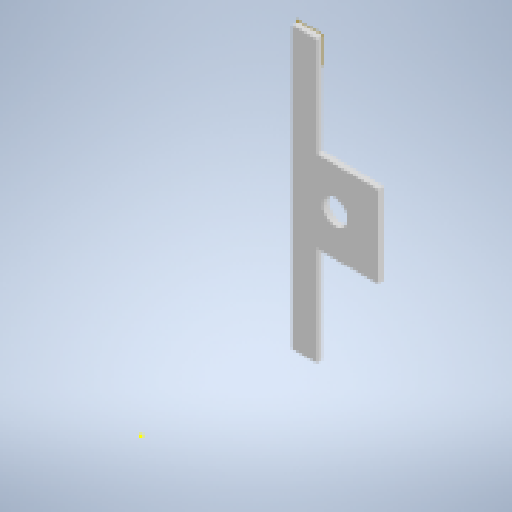
# Autodesk Inventor part: Linear rod connecting plate
Saved by Autodesk Inventor 2023.1 (Build 271208000, 208)
## iProperties
Created: 2023-02-01
Part Number: Linear rod connecting plate
Material: Generic
Document SubType Name: Modeling
Designer: dmargari
Density: 1 g/cm^3
Appearance: Default
Author: dmargari
Autodesk Inventor part; units mm, degrees
ref_plane "YZ Plane" through (0, 0, 0) normal (1, 0, 0) x (0, 1, 0)
ref_plane "XZ Plane" through (0, 0, 0) normal (0, 1, 0) x (-1, 0, 0)
ref_plane "XY Plane" through (0, 0, 0) normal (0, 0, 1) x (1, 0, 0)
sketch "Sketch1" plane through (0, 0, 0) normal (0, 0, 1) x (1, 0, 0)
  point P0 (0, 0)
ref_plane "Work Plane1" through (0, 125.1054, -82.3097) normal (0, 0, 1) x (1, 0, 0)
sketch "Sketch2" plane through (0, 125.1054, -82.3097) normal (0, 0, 1) x (1, 0, 0)
  circle A0 centre (0.3907, 0.2373) radius 6 projected
  circle A1 centre (0.3907, -124.7627) radius 6 projected
  line L0 (6.3907, 6.2373) -> (-5.6093, 6.2373)
  line L1 (-5.6093, 6.2373) -> (-5.6093, -130.7627)
  line L2 (-5.6093, -130.7627) -> (6.3907, -130.7627)
  line L3 (6.3907, -130.7627) -> (6.3907, 6.2373)
  point P0 (0, -125.1054)
  constraints: 8 end point, 2 parallel, 2 tangent, 1 horizontal, 1 perpendicular
extrude "Extrusion1" add sketch "Sketch2" along normal blind 3
sketch "Sketch5" plane through (6.3907, -5.6573, -82.3097) normal (1, 0, 0) x (0, 0, -1)
  line L0 (0, 0) -> (0, 137) projected
  line L1 (0, 137) -> (-3, 137) projected
  line L2 (-3, 0) -> (-3, 137) projected
  line L3 (0, 0) -> (-3, 0) projected
  line L4 (-3, 0) -> (-3, 137) construction
  line L5 (-3, 68.5) -> (0, 68.5) construction
  line L6 (0, 0) -> (0, 137) construction
  line L7 (-3, 48.5) -> (0, 48.5)
  line L8 (0, 48.5) -> (0, 88.5)
  line L9 (0, 88.5) -> (-3, 88.5)
  line L10 (-3, 88.5) -> (-3, 48.5)
  line L11 (-3, 48.5) -> (0, 88.5) construction
  line L12 (0, 48.5) -> (-3, 88.5) construction
  point P0 (-82.3097, 5.6573)
  point P1 (-1.5, 68.5)
  point P2 (0, 88.5)
  point P3 (-3, 88.5)
  point P4 (-3, 48.5)
  point P5 (0, 48.5)
  dimension "d9" = 3
  dimension "d10" = 40
  constraints: 14 end point, 5 midpoint, 2 parallel, 1 horizontal, 1 perpendicular
  measures "d9" distance of L9.end L8.end
  measures "d10" distance of L8.end L7.end
extrude "Extrusion4" add sketch "Sketch5" along normal blind 30 contours L7 L2 L9 L0
sketch "Sketch6" plane through (0, 125.1054, -82.3097) normal (0, 0, -1) x (-1, 0, 0)
  point P0 (0, -125.1054)
sketch "Sketch7" plane through (0, 125.1054, -79.3097) normal (0, 0, 1) x (1, 0, 0)
  line L0 (6.3907, 6.2373) -> (-5.6093, 6.2373) construction
  line L1 (-5.6093, 6.2373) -> (-5.6093, -130.7627) construction
  line L2 (-5.6093, -130.7627) -> (6.3907, -130.7627) construction
  line L3 (6.3907, -130.7627) -> (6.3907, -82.2627) construction
  line L4 (6.3907, -82.2627) -> (36.3907, -82.2627) construction
  line L5 (36.3907, -42.2627) -> (36.3907, -82.2627) construction
  line L6 (6.3907, -42.2627) -> (36.3907, -42.2627) construction
  line L7 (6.3907, -42.2627) -> (6.3907, 6.2373) construction
  line L8 (6.3907, -130.7627) -> (6.3907, -82.2627) construction
  line L9 (6.3907, -42.2627) -> (6.3907, -82.2627) construction
  circle A0 centre (15.3907, -62.2627) radius 6
  point P0 (0, -125.1054)
  point P1 (6.3907, -62.2627)
  dimension "d13" = 12
  dimension "d14" = 9
  constraints: 2 end point, 1 centre point, 1 midpoint, 1 vertical
  measures "d13" diameter of A0
  measures "d14" distance of point (6.391, -62.263) A0.centre
extrude "Extrusion5" cut sketch "Sketch7" against normal blind 30
body "Solid1"
